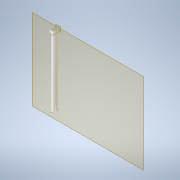
# Autodesk Inventor part: Riegel1
Saved by Autodesk Inventor 2021.3 (Build 253353010, 353A)
## iProperties
Created: 2021-08-03
Part Number: Riegel1
Material: Generisch
Document SubType Name: Modeling
Designer: Markus
Density: 1 g/cm^3
Appearance: Vorgabe
Author: Markus
Autodesk Inventor part; units mm, degrees
ref_plane "YZ Plane" through (0, 0, 0) normal (1, 0, 0) x (0, 1, 0)
ref_plane "XZ Plane" through (0, 0, 0) normal (0, 1, 0) x (-1, 0, 0)
ref_plane "XY Plane" through (0, 0, 0) normal (0, 0, 1) x (1, 0, 0)
ref_plane "Arbeitsebene1" through (38, 35.4, -7.95) normal (0, 0, -1) x (-1, 0, 0)
ref_plane "Arbeitsebene2" through (0, 0, 0) normal (0, 0, 1) x (1, 0, 0)
sketch "Skizze2" plane through (0, 0, 0) normal (0, 0, 1) x (1, 0, 0)
  arc A0 (16, 69.8) -> (15, 70.8) centre (15, 69.8) ccw projected
  line L0 (15, 70.8) -> (1.5128, 70.8) projected
  arc A1 (1.0229, 71.2002) -> (1.5128, 70.8) centre (1.5128, 71.3) ccw projected
  arc A2 (1.0229, 71.2002) -> (-4.1832, 67.0287) centre (-2.6517, 70.4517) ccw projected
  arc A3 (-3, 65.2031) -> (-4.1832, 67.0287) centre (-5, 65.2031) ccw projected
  line L1 (-3, 65.2031) -> (-3, 2) projected
  arc A4 (-3, 2) -> (-1, 0) centre (-1, 2) ccw projected
  line L2 (-1, 0) -> (3, 0) projected
  line L3 (3, 0) -> (3, 3) projected
  line L4 (3, 3) -> (0.3, 3) projected
  arc A5 (0, 3.3) -> (0.3, 3) centre (0.3, 3.3) ccw projected
  line L5 (0, 3.3) -> (0, 67.5) projected
  arc A6 (0.3, 67.8) -> (0, 67.5) centre (0.3, 67.5) ccw projected
  line L6 (0.3, 67.8) -> (15, 67.8) projected
  arc A7 (15, 67.8) -> (16, 68.8) centre (15, 68.8) ccw projected
  line L7 (16, 68.8) -> (16, 69.8) projected
  circle A8 centre (-2.6517, 70.4517) radius 1.25 projected
  line L8 (1.5128, 70.8) -> (4.3, 70.8) projected
  line L9 (4.3, 67.8) -> (0.3, 67.8) projected
  arc A9 (4, 68.1) -> (4.3, 67.8) centre (4.3, 68.1) ccw projected
  line L10 (4, 70.5) -> (4, 68.1) projected
  arc A10 (4.3, 70.8) -> (4, 70.5) centre (4.3, 70.5) ccw projected
  line L11 (1.5128, 70.8) -> (4.3, 70.8) projected
  arc A11 (1.0229, 71.2002) -> (1.5128, 70.8) centre (1.5128, 71.3) ccw projected
  arc A12 (1.0229, 71.2002) -> (-0.0955, 73.1955) centre (-2.6517, 70.4517) ccw projected
  arc A13 (0, 72.976) -> (-0.0955, 73.1955) centre (-0.3, 72.976) ccw projected
  line L12 (0, 72.976) -> (0, 67.5) projected
  arc A14 (0.3, 67.8) -> (0, 67.5) centre (0.3, 67.5) ccw projected
  line L13 (4, 70.8) -> (4, 73.8)
  line L14 (4, 73.8) -> (-0.9631, 73.8)
  point P0 (0, 0)
  dimension "d1" = 3
  constraints: 4 end point, 1 collinear, 1 perpendicular, 1 point on circle, 1 point on line
  measures "d1" distance of L13.start L13.end
extrude "Extrusion1" add sketch "Skizze2" against normal mid plane 5 contours L0 A1 A2 L14 L13
ref_plane "Arbeitsebene3" through (1.5128, 70.8, -2.5) normal (0, -1, 0) x (1, 0, 0)
sketch "Skizze3" plane through (1.5128, 70.8, -2.5) normal (0, -1, 0) x (1, 0, 0)
  line L0 (2.4872, 4.75) -> (2.7872, 4.75) projected
  line L1 (-1.2128, 0.25) -> (-1.5128, 0.25) projected
  line L2 (-1.2128, 4.75) -> (2.7872, 4.75) projected
  line L3 (0, 0) -> (0, 5) projected
  line L4 (2.4872, 0) -> (0, 0) projected
  line L5 (2.4872, 0) -> (2.4872, 5) projected
  line L6 (0, 5) -> (2.4872, 5) projected
  line L7 (0, 0) -> (0, 5) projected
  line L8 (0, 0.25) -> (0, 4.75)
  line L9 (0, 4.75) -> (2.4872, 4.75)
  line L10 (2.4872, 0) -> (2.4872, 5) projected
  line L11 (2.4872, 0.25) -> (2.4872, 4.75)
  line L12 (2.7872, 0.25) -> (-1.5128, 0.25) projected
  line L13 (0, 0.25) -> (2.4872, 0.25)
  line L14 (0.1, 4.65) -> (2.4872, 4.65)
  line L15 (2.4872, 4.65) -> (2.4872, 0.35)
  line L16 (2.4872, 0.35) -> (0.1, 0.35)
  line L17 (0.1, 0.35) -> (0.1, 4.65)
  point P0 (0.1, 2.5)
  point P1 (0, 2.5)
  point P2 (1.2436, 4.75)
  point P3 (2.4872, 2.5)
  dimension "d6" = 0.1
  dimension "d28" = 0.1
  constraints: 16 end point, 5 midpoint, 4 point on line, 3 perpendicular, 2 collinear, 2 parallel, 1 horizontal, 1 horizontal alignment
  measures "d6" distance between parallel lines of L9 L14
  measures "d28" distance between parallel lines of L8 L17
extrude "Extrusion2" add sketch "Skizze3" along normal blind 72 contours L5 L16 L17 L14
sketch "Skizze4" plane through (4, -1.2, 2.15) normal (1, 0, 0) x (0, 0, -1)
  line L0 (0, 72) -> (0, 0) projected
  line L1 (4.3, 0) -> (0, 0) projected
  line L2 (4.3, 72) -> (4.3, 0) projected
  line L3 (-1.5, 1) -> (5.8, 1)
  line L4 (0, 0) -> (4.3, 0) projected
  line L5 (3.8, 0) -> (0.5, 0)
  line L6 (3.8, 0) -> (5.8, 1)
  line L7 (0.5, 0) -> (-1.5, 1)
  line L8 (2.15, -15) -> (2.15, 90) projected
  line L9 (4.4, 1.2) -> (-0.1, 1.2) projected
  point P0 (0, 1)
  point P1 (2.15, 0)
  point P2 (0, 0.25)
  dimension "d10" = 1.5
  dimension "d13" = 1.5
  dimension "d22" = 0.5
  dimension "d23" = 0.2
  constraints: 8 end point, 3 point on line, 1 horizontal, 1 midpoint
  measures "d10" distance from line of L0 L3.start
  measures "d13" distance from line of L2 L3.end
  measures "d22" distance from line of L2 L5.start
  measures "d23" distance between parallel lines of L9 L3
extrude "Extrusion3" add sketch "Skizze4" against normal up to surface (2.3872 mm away) contours L3 L8 L1 L7 L0 | L0 L7 L3 | L7 L1 L0 | L3 L2 L6 L1 L8 | L3 L6 L2
sketch "Skizze5" plane through (4, 70.8, 2.15) normal (1, 0, 0) x (0, 0, 1)
  line L0 (-4.3, 72) -> (0, 72) projected
  line L1 (0, 0) -> (0, 71) projected
  line L2 (-4.3, 0) -> (-4.3, 71) projected
  line L3 (-3.65, 72) -> (-0.65, 72)
  line L4 (-3.65, 72) -> (-2.15, 65)
  line L5 (-2.15, 65) -> (-0.65, 72)
  arc A0 (-2.2548, 65.4889) -> (-2.0452, 65.4889) centre (-2.15, 65) ccw
  point P0 (-2.15, 70.8)
  point P1 (4.3, -73)
  point P2 (0, -73)
  point P3 (0, -71.7017)
  point P4 (4.3, -71.7017)
  point P5 (-2.15, 72)
  point P6 (-2.15, 72)
  point P7 (-2.2207, 65.495)
  point P8 (-2.0793, 65.495)
  dimension "d16" = 3
  dimension "d18" = 1
  dimension "d29" = 7
  constraints: 6 end point, 2 point on circle, 2 point on line, 1 centre point, 1 coincident, 1 midpoint, 1 vertical alignment, 6 other
  measures "d16" distance of L3.end L3.start
  measures "d18" diameter of A0
  measures "d29" vertical distance of L3.start L4.end
extrude "Extrusion4" cut sketch "Skizze5" against normal up to next
fillet "Rundung1" radius 0.1 4 edges at (2.8064, -0.2, -3.65) (2.8064, -0.2, 3.65) (2.8064, 5.3111, -0.1048) (2.8064, 5.3111, 0.1048)
fillet "Rundung2" radius 0.5 4 edges at (2.8064, -1.2, 2.15) (2.8064, -1.2, -1.5) (2.8064, -1.2, 1.5) (2.8064, -1.2, -2.15)
fillet "Rundung3" radius 0.2 2 edges at (2.8064, -0.2, -2.15) (2.8064, -0.2, 2.15)
fillet "Rundung4" radius 0.2 8 edges at (1.5184, 73.8, 2.5) (4, 73.8, 0) (1.5184, 73.8, -2.5) (-0.9631, 73.8, 0) (1.1965, 70.9128, 2.5) (0.3283, 72.7281, 2.5) (2.7564, 70.8, 2.5) (4, 72.3, -2.5)
equation "\"d28\" = d6"
equation "\"d13\" = d10"
equation "\"d16\" = 2 * d10"
